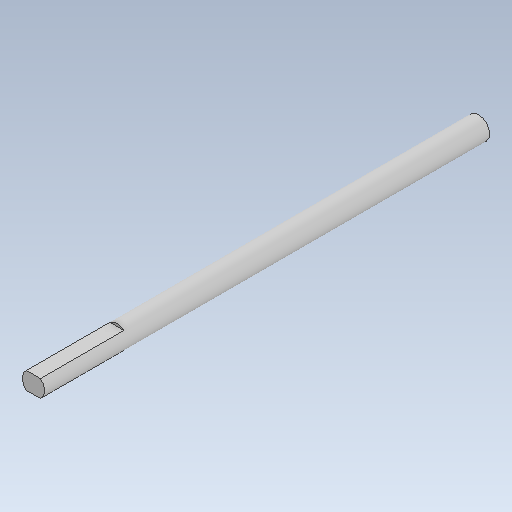
# Autodesk Inventor part: oś napędowa
Saved by Autodesk Inventor 2021 (Build 250183000, 183)
## iProperties
Created: 2021-06-27
Part Number: oś napędowa
Material: Generic
Document SubType Name: Modeling
Designer: Łukasz
Density: 1 g/cm^3
Appearance: Default
Author: Łukasz
Autodesk Inventor part; units mm, degrees
ref_plane "YZ Plane" through (0, 0, 0) normal (1, 0, 0) x (0, 1, 0)
ref_plane "XZ Plane" through (0, 0, 0) normal (0, 1, 0) x (-1, 0, 0)
ref_plane "XY Plane" through (0, 0, 0) normal (0, 0, 1) x (1, 0, 0)
sketch "Sketch1" plane through (0, 0, 0) normal (0, 0, 1) x (1, 0, 0)
  circle A0 centre (0, 0) radius 4
  dimension "d0" = 8
  constraints: 1 centre point, 1 coincident
  measures "d0" diameter of A0
extrude "Extrusion1" add sketch "Sketch1" along normal blind 160
sketch "Sketch2" plane through (0, 0, 160) normal (0, 0, 1) x (1, 0, 0)
  line L0 (-2.5278, 3.1) -> (2.5278, 3.1)
  line L1 (2.5278, -3.1) -> (-2.5278, -3.1)
  arc A0 (-2.5278, 3.1) -> (-2.5278, -3.1) centre (0, 0) ccw
  arc A1 (2.5278, -3.1) -> (2.5278, 3.1) centre (0, 0) ccw
  line L2 (-2.5278, 3.1) -> (3.1486, 3.1)
  line L3 (3.1486, 3.1) -> (3.1486, 5.5336)
  line L4 (3.1486, 5.5336) -> (-2.5278, 5.5336)
  line L5 (-2.5278, 5.5336) -> (-2.5278, 3.1)
  line L6 (2.5278, -3.1) -> (-2.7681, -3.1)
  line L7 (-2.7681, -3.1) -> (-2.7681, -5.0994)
  line L8 (-2.7681, -5.0994) -> (2.5278, -5.0994)
  line L9 (2.5278, -5.0994) -> (2.5278, -3.1)
  dimension "d3" = 3.1
  constraints: 20 end point, 5 parallel, 4 point on circle, 3 coincident, 3 horizontal, 2 centre point, 2 perpendicular
  measures "d3" distance from line of point (0, 0) L0
extrude "Extrusion2" cut sketch "Sketch2" against normal blind 30 contours L5 L4 L3 L2 L0 | L1 L9 L8 L7 L6
body "Solid1"
